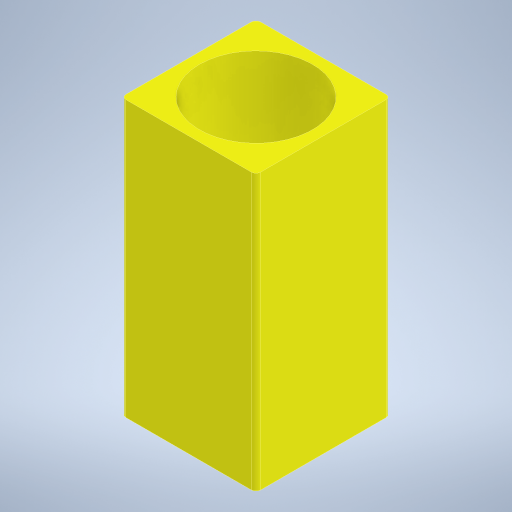
# Autodesk Inventor part: Sulfur_electrode
Saved by Autodesk Inventor 2023 (Build 270158000, 158)
## iProperties
Created: 2022-09-21
Part Number: Sulfur_electrode
Material: ПВХ, гибкий
Document SubType Name: Modeling
Designer: Makar
Density: 2.07 g/cm^3
Appearance: Желтый
Mass: 160.005 g
Surface Area: 277.875 cm^2
Volume: 77.2973 cm^3
Author: Makar
Autodesk Inventor part; units mm, degrees
ref_plane "YZ Plane" through (0, 0, 0) normal (1, 0, 0) x (0, 1, 0)
ref_plane "XZ Plane" through (0, 0, 0) normal (0, 1, 0) x (-1, 0, 0)
ref_plane "XY Plane" through (0, 0, 0) normal (0, 0, 1) x (1, 0, 0)
sketch "Эскиз1" plane through (0, 0, 0) normal (0, 1, 0) x (-1, 0, 0)
  circle A0 centre (20.5, 24) radius 18.5
  line L0 (42.5, 44.5) -> (42.5, 3.5)
  line L1 (0, 46) -> (41, 46)
  arc A1 (42.5, 44.5) -> (41, 46) centre (41, 44.5) ccw
  arc A2 (0, 46) -> (-1.5, 44.5) centre (0, 44.5) ccw
  line L2 (-1.5, 3.5) -> (-1.5, 44.5)
  arc A3 (-1.5, 3.5) -> (0, 2) centre (0, 3.5) ccw
  line L3 (41, 2) -> (0, 2)
  arc A4 (41, 2) -> (42.5, 3.5) centre (41, 3.5) ccw
  point P0 (0, 0)
  constraints: 8 end point, 8 point on circle, 5 centre point
extrude "Выдавливание1" add sketch "Эскиз1" along normal blind 90
